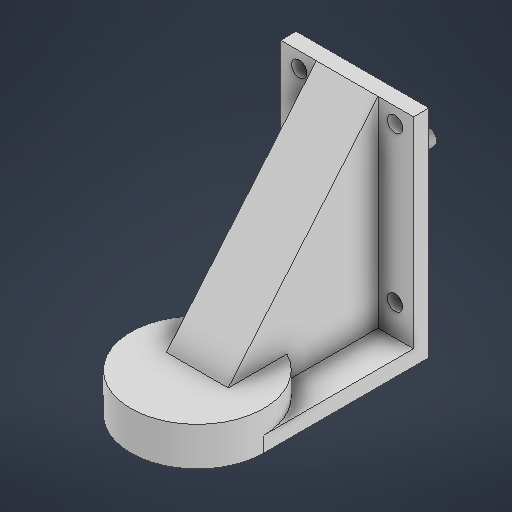
# Autodesk Inventor part: Dam1
Saved by Autodesk Inventor 2027 (Build 310192060, 192F)
## iProperties
Created: 2026-08-17
Part Number: Dam1
Material: Generic
Document SubType Name: Modeling
Designer: trtrn
Density: 1 g/cm^3
Appearance: Default
Author: trtrn
Autodesk Inventor part; units mm, degrees
ref_plane "YZ Plane" through (0, 0, 0) normal (1, 0, 0) x (0, 1, 0)
ref_plane "XZ Plane" through (0, 0, 0) normal (0, 1, 0) x (-1, 0, 0)
ref_plane "XY Plane" through (0, 0, 0) normal (0, 0, 1) x (1, 0, 0)
sketch "Sketch1" plane through (0, 0, 0) normal (0, 0, 1) x (1, 0, 0)
  line L0 (-21.5, 35) -> (21.5, 35)
  line L1 (21.5, 35) -> (21.5, -35)
  line L2 (21.5, -35) -> (-21.5, -35)
  line L3 (-21.5, -35) -> (-21.5, 35)
  line L4 (-21.5, 35) -> (21.5, -35) construction
  line L5 (21.5, 35) -> (-21.5, -35) construction
  point P0 (0, 0)
  dimension "d0" = 43
  dimension "d1" = 70
  constraints: 12 end point, 2 midpoint, 2 parallel, 1 horizontal, 1 perpendicular
  measures "d0" distance of L1.end L2.end
  measures "d1" distance of L0.end L1.end
extrude "Extrusion1" add sketch "Sketch1" along normal blind 5
sketch "Sketch3" plane through (0, 0, 5) normal (0, 0, 1) x (1, 0, 0)
  line L0 (-21.5, 35) -> (-21.5, -35) projected
  line L1 (-21.5, -35) -> (21.5, -35) projected
  line L2 (21.5, -35) -> (21.5, 35) projected
  line L3 (-21.5, -30) -> (21.5, -30)
  line L4 (21.5, -30) -> (21.5, -35)
  line L5 (21.5, -35) -> (-21.5, -35)
  line L6 (-21.5, -35) -> (-21.5, -30)
  point P0 (0, 0)
  dimension "d5" = 5
  constraints: 8 end point, 2 parallel, 1 horizontal, 1 perpendicular, 1 point on line
  measures "d5" distance between parallel lines of L1 L3
extrude "Extrusion2" add sketch "Sketch3" along normal blind 70
sketch "Sketch4" plane through (-21.5, -30, 5) normal (0, 1, 0) x (1, 0, 0)
  line L0 (43, 0) -> (43, -70) projected
  line L1 (43, -70) -> (0, -70) projected
  line L2 (0, 0) -> (0, -70) projected
  arc A0 (0, -48.5) -> (43, -48.5) centre (21.5, -48.5) ccw
  line L3 (0, -70) -> (43, -70) projected
  line L4 (21.5, -70) -> (43, -70)
  line L5 (43, -70) -> (43, -48.5)
  line L6 (43, 5) -> (43, -70) projected
  line L7 (0, 5) -> (0, -70) projected
  line L8 (0, -48.5) -> (0, -70)
  line L9 (0, -70) -> (21.5, -70)
  circle A1 centre (21.5, -48.5) radius 18.5
  point P0 (21.5, 5)
  point P1 (0, -48.5)
  dimension "d10" = 37
  constraints: 8 end point, 4 tangent, 3 point on circle, 2 centre point, 2 point on line, 1 coincident, 1 collinear, 1 midpoint, 1 perpendicular, 1 vertical
  measures "d10" diameter of A1
extrude "Extrusion5" cut sketch "Sketch4" against normal blind 100 contours L1 L2 A0 | L0 L1 A0
extrude "Extrusion6" cut sketch "Sketch4" against normal blind 100 contours A1
sketch "Sketch5" plane through (0, 0, 5) normal (0, 0, 1) x (1, 0, 0)
  line L0 (0, -49) -> (0, 49) projected
  line L1 (21.5, 35) -> (-21.5, 35) projected
  point P0 (0, 0)
  point P1 (-15.5, 30)
  point P2 (15.5, 30)
  point P3 (15.5, 21)
  point P4 (-15.5, -20)
  point P5 (15.5, -20)
  point P6 (-15.5, -11)
  dimension "d17" = 31
  dimension "d18" = 5
  dimension "d19" = 9
  dimension "d20" = 50
  dimension "d21" = 9
  constraints: 4 vertical alignment, 1 horizontal alignment, 1 symmetric about line
  measures "d17" distance of point (15.5, 30) point (-15.5, 30)
  measures "d18" distance from line of point (-15.5, 30) L1
  measures "d19" distance of point (15.5, 21) point (15.5, 30)
  measures "d20" distance of point (15.5, -20) point (15.5, 30)
  measures "d21" distance of point (-15.5, -11) point (-15.5, -20)
hole "Hole1" at (-15.5, 30, 5) at (15.5, 30, 5) at (15.5, 21, 5) at (-15.5, -20, 5) at (15.5, -20, 5) at (-15.5, -11, 5) direction (0, 0, -1) diameter 5 end through all
sketch "Sketch6" plane through (0, 0, 5) normal (0, 0, 1) x (1, 0, 0)
  circle A0 centre (15.5, 21) radius 2.5 projected
  circle A1 centre (15.5, 21) radius 2.5
  circle A2 centre (-15.5, -11) radius 2.5 projected
  circle A3 centre (-15.5, -11) radius 2.5
  point P0 (0, 0)
  constraints: 2 centre point, 2 coincident
extrude "Extrusion7" add sketch "Sketch6" against normal blind 11
sketch "Sketch7" plane through (0, 0, 5) normal (0, 0, 1) x (1, 0, 0)
  line L0 (21.5, 35) -> (-21.5, 35) projected
  line L1 (-18.5, -30) -> (18.5, -30) projected
  line L2 (-10, 35) -> (10, 35)
  line L3 (10, 35) -> (10, -30)
  line L4 (10, -30) -> (-10, -30)
  line L5 (-10, -30) -> (-10, 35)
  line L6 (0, -49) -> (0, 49) projected
  point P0 (0, 0)
  dimension "d31" = 20
  constraints: 8 end point, 2 parallel, 2 point on line, 1 horizontal, 1 perpendicular, 1 other
  measures "d31" distance between parallel lines of L5 L3
extrude "Extrusion8" add sketch "Sketch7" along normal blind 48.5
sketch "Sketch12" plane through (0, -30, 53.5) normal (0, 1, 0) x (1, 0, 0)
  line L0 (-10, 0) -> (10, 0) projected
  circle A0 centre (0, 0) radius 21.5
  arc A1 (-21.5, 0) -> (21.5, 0) centre (0, 0) ccw projected
  point P0 (0, 53.5)
  constraints: 2 concentric, 1 centre point, 1 midpoint
extrude "Extrusion13" add sketch "Sketch12" along normal blind 7.5
sketch "Sketch13" plane through (-10, -30, 5) normal (-1, 0, 0) x (0, 0, 1)
  line L0 (-5, 65) -> (0, 65) projected
  line L1 (48.5, 7.5) -> (48.5, 65) projected
  line L2 (0, 65) -> (48.5, 7.5)
  line L3 (48.5, 7.5) -> (48.5, 65)
  line L4 (48.5, 65) -> (0, 65)
  point P0 (-5, 30)
  constraints: 6 end point, 1 collinear, 1 perpendicular
extrude "Extrusion14" cut sketch "Sketch13" against normal blind 48.5
body "Solid1"
